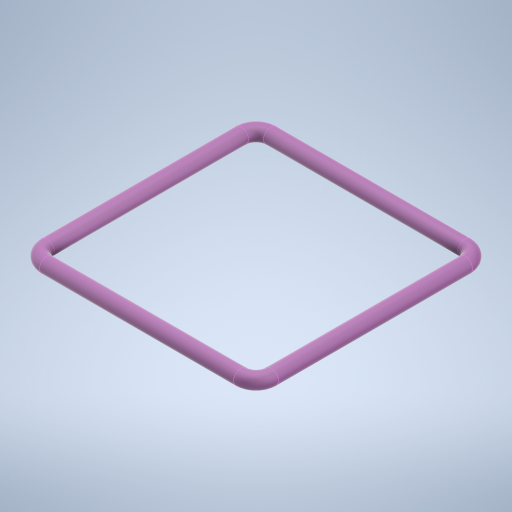
# Autodesk Inventor part: Pool Noodles
Saved by Autodesk Inventor 2023 (Build 270158000, 158)
## iProperties
Created: 2023-11-22
Part Number: Pool Noodles
Material: Generic
Document SubType Name: Modeling
Designer: adamarnold
Density: 1 g/cm^3
Appearance: Smooth - Purple
Author: adamarnold
Autodesk Inventor part; units mm, degrees
ref_plane "XZ Plane" through (0, 0, 0) normal (0, 1, 0) x (-1, 0, 0)
ref_plane "XY Plane" through (0, 0, 0) normal (0, 0, 1) x (1, 0, 0)
sketch "Sketch1" plane through (0, 0, 0) normal (0, 1, 0) x (-1, 0, 0)
  line L0 (50.8, 0) -> (708.025, 0)
  line L1 (758.825, -50.8) -> (758.825, -708.025)
  line L2 (708.025, -758.825) -> (50.8, -758.825)
  line L3 (0, -708.025) -> (0, -50.8)
  arc A0 (758.825, -50.8) -> (708.025, 0) centre (708.025, -50.8) ccw
  arc A1 (708.025, -758.825) -> (758.825, -708.025) centre (708.025, -708.025) ccw
  arc A2 (0, -708.025) -> (50.8, -758.825) centre (50.8, -708.025) ccw
  arc A3 (50.8, 0) -> (0, -50.8) centre (50.8, -50.8) ccw
  point P0 (0, 0)
  point P1 (758.825, -758.825)
  point P2 (758.825, 0)
  point P3 (0, -758.825)
  dimension "d0" = 758.825
  dimension "d1" = 758.825
  dimension "d2" = 50.8
  constraints: 8 end point, 8 point on circle, 8 point on line, 8 tangent, 4 centre point, 3 equal radius, 2 parallel, 1 horizontal, 1 perpendicular
  measures "d0" distance of point (758.825, -758.825) point (0, -758.825)
  measures "d1" distance of point (758.825, 0) point (758.825, -758.825)
  measures "d2" radius of A0
ref_plane "Work Plane1" through (-379.4125, 0, 0) normal (1, 0, 0) x (0, 1, 0)
sketch "Sketch2" plane through (-379.4125, 0, 0) normal (1, 0, 0) x (0, 1, 0)
  circle A0 centre (0, 0) radius 25.4
  dimension "d4" = 50.8
  constraints: 1 centre point, 1 coincident
  measures "d4" diameter of A0
sweep "Sweep1" add profiles "Sketch2" path "Sketch1" path curves L0 A0 L1 A1 L2 A2 L3 A3
body "Solid1"
